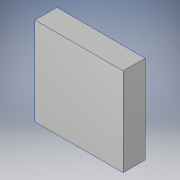
# Autodesk Inventor part: al
Saved by Autodesk Inventor 2019 (Build 230136000, 136)
## iProperties
Created: 2021-07-12
Part Number: al
Material: Generic
Document SubType Name: Modeling
Designer: pensun
Density: 1 g/cm^3
Appearance: Default
Author: pensun
Autodesk Inventor part; units mm, degrees
ref_plane "YZ Plane" through (0, 0, 0) normal (1, 0, 0) x (0, 1, 0)
ref_plane "XZ Plane" through (0, 0, 0) normal (0, 1, 0) x (-1, 0, 0)
ref_plane "XY Plane" through (0, 0, 0) normal (0, 0, 1) x (1, 0, 0)
sketch "Sketch1" plane through (0, 0, 0) normal (0, 0, 1) x (1, 0, 0)
  line L0 (-20, 20) -> (20, 20)
  line L1 (20, 20) -> (20, -20)
  line L2 (20, -20) -> (-20, -20)
  line L3 (-20, -20) -> (-20, 20)
  point P0 (0, 0)
  dimension "d1" = 20
  dimension "d2" = 40
  dimension "d3" = 40
  dimension "d4" = 20
  constraints: 8 end point, 2 parallel, 1 horizontal, 1 perpendicular
  measures "d1" distance from line of L1 point (0, 0)
  measures "d2" distance of L1.end L2.end
  measures "d3" distance of L2.end L0.start
  measures "d4" distance from line of L2 point (0, 0)
extrude "Extrusion1" add sketch "Sketch1" along normal blind 10
body "Solid1"
